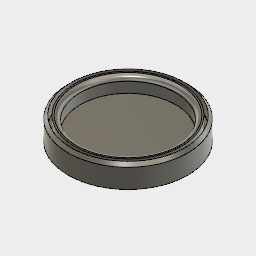
ANS0016_static_top v2 (Autodesk Fusion 360 design; units mm, degrees)
Autodesk Fusion 360 part; units mm, degrees
sketch "Sketch1" plane through (0, 0, 0) normal (0, 1, 0) x (1, 0, 0)
  circle A0 centre (0, 0) radius 40
  dimension "d1" = 80
  measures "d1" diameter of A0
extrude "Extrude1" add sketch "Sketch1" along normal blind 15
sketch "Sketch2" plane through (0, 15, 0) normal (0, 1, 0) x (-1, 0, 0)
  circle A0 centre (0, 0) radius 40
  circle A1 centre (0, 0) radius 38
  circle A2 centre (0, 0) radius 36
  dimension "d4" = 76
  dimension "d5" = 72
  measures "d4" diameter of A1
  measures "d5" diameter of A2
extrude "Extrude2" cut sketch "Sketch2" against normal blind 8 contours A1
chamfer "Chamfer1" distance 2 angle 45 1 edges at (-37.2931, 15, 14.4646)
sketch "Sketch3" plane through (0, 15, 0) normal (0, 1, 0) x (-1, 0, 0)
  circle A0 centre (0, 0) radius 36
  circle A1 centre (0, 0) radius 32
  dimension "d9" = 64
  measures "d9" diameter of A1
extrude "Extrude3" cut sketch "Sketch3" against normal blind 10 contours A1
fillet "Fillet1" radius 3 1 edges at (29.8345, 15, 11.5717)
